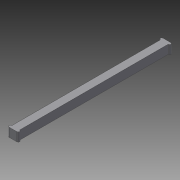
# Autodesk Inventor part: Arrow_Shaft_Template
Saved by Autodesk Inventor 2014 (Build 180170000, 170)
## iProperties
Created: 2014-10-19
Part Number: Arrow_Shaft_Template
Material: Generic
Document SubType Name: Modeling
Designer: ThatOtherGuy
Density: 1 g/cm^3
Appearance: Default
Author: ThatOtherGuy
Autodesk Inventor part; units mm, degrees
ref_plane "YZ Plane" through (0, 0, 0) normal (1, 0, 0) x (0, 1, 0)
ref_plane "XZ Plane" through (0, 0, 0) normal (0, 1, 0) x (-1, 0, 0)
ref_plane "XY Plane" through (0, 0, 0) normal (0, 0, 1) x (1, 0, 0)
sketch "Sketch1" plane through (0, 0, 0) normal (0, 0, 1) x (1, 0, 0)
  line L0 (0, 0) -> (8.75, 0)
  line L1 (8.75, 0) -> (8.75, 175)
  line L2 (8.75, 175) -> (0, 175)
  line L3 (0, 175) -> (0, 0)
  arc A0 (0, 3.175) -> (0, 0) centre (0, 1.5875) ccw
  arc A1 (8.75, 0) -> (8.75, 3.175) centre (8.75, 1.5875) ccw
  arc A2 (0, 175) -> (0, 171.825) centre (0, 173.4125) ccw
  arc A3 (8.75, 171.825) -> (8.75, 175) centre (8.75, 173.4125) ccw
  dimension "d0" = 8.75
  dimension "d1" = 175
  dimension "d2" = 1.5875
  constraints: 8 end point, 8 point on circle, 4 centre point, 4 point on line, 4 tangent, 3 equal radius, 2 parallel, 1 horizontal, 1 perpendicular
  measures "d0" distance of L0.start L0.end
  measures "d1" distance of L2.end L0.start
  measures "d2" radius of A0
extrude "Extrusion1" add sketch "Sketch1" along normal blind 10
body "Solid1"
